DHECsensorcase (Autodesk Fusion 360 design; units mm, degrees)
Autodesk Fusion 360 part; units mm, degrees
sketch "Sketch1" plane through (0, 0, 0) normal (0, 0, 1) x (1, 0, 0)
  line L0 (0, 0) -> (50, 0)
  line L1 (50, 0) -> (50, 39)
  line L2 (50, 39) -> (0, 39)
  line L3 (0, 39) -> (0, 0)
  line L4 (2, 2) -> (48, 2)
  line L5 (48, 2) -> (48, 37)
  line L6 (48, 37) -> (2, 37)
  line L7 (2, 37) -> (2, 2)
  dimension "d1" = 46
  dimension "d2" = 2
  dimension "d3" = 2
  dimension "d4" = 2
  dimension "d5" = 2
  dimension "d6" = 35
  constraint horizontal L0
  constraint vertical L1
  constraint horizontal L2
  constraint vertical L3
  constraint coincident L0.start L3.end
  constraint horizontal L4
  constraint vertical L5
  constraint horizontal L6
  constraint vertical L7
  measures "d1" distance of L5 L7
  measures "d2" distance of L3 L7
  measures "d3" distance of L2 L6
  measures "d4" distance of L0 L4
  measures "d5" distance of L1 L5
  measures "d6" distance of L4 L6
extrude "Extrude1" add sketch "Sketch1" along normal blind 2 contours L4 L5 L6 L7
extrude "Extrude2" add sketch "Sketch1" along normal blind 25
sketch "Sketch2" plane through (50, 0, 0) normal (1, 0, 0) x (0, 1, 0)
  line L0 (0, 0) -> (39, 0)
  line L1 (39, 0) -> (39, 25)
  line L2 (39, 25) -> (0, 25)
  line L3 (0, 25) -> (0, 0)
  line L4 (2, 25) -> (2, 24)
  line L5 (2, 24) -> (1, 24)
  line L6 (1, 24) -> (1, 23)
  line L7 (1, 23) -> (38, 23)
  line L8 (38, 23) -> (38, 24)
  line L9 (38, 24) -> (37, 24)
  line L10 (37, 24) -> (37, 25)
  line L11 (2, 23) -> (37, 23)
  line L12 (37, 23) -> (37, 4)
  line L13 (37, 4) -> (2, 4)
  line L14 (2, 4) -> (2, 23)
  dimension "d11" = 1
  dimension "d12" = 1
  dimension "d13" = 1
  dimension "d14" = 1
  dimension "d15" = 1
  dimension "d16" = 1
  dimension "d17" = 1
  dimension "d18" = 19
  constraint coincident L2 L4.start
  constraint perpendicular L2 L4
  constraint perpendicular L4 L5
  constraint perpendicular L2 L6
  constraint perpendicular L6 L7
  constraint perpendicular L7 L8
  constraint perpendicular L6 L9
  constraint coincident L2 L10.end
  constraint perpendicular L2 L10
  constraint horizontal L11
  constraint vertical L12
  constraint horizontal L13
  constraint vertical L14
  constraint coincident L7 L11.start
  constraint coincident L4.end L14
  constraint coincident L9.end L12
  measures "d11" distance of L2 L5
  measures "d12" distance of L5 L7
  measures "d13" distance of L4 L6
  measures "d14" distance of L3 L6
  measures "d15" distance of L1 L8
  measures "d16" distance of L8 L10
  measures "d17" distance of L7 L9
  measures "d18" distance of L11 L13
extrude "Extrude3" cut sketch "Sketch2" against normal up to surface (48 mm away) contours L2 L4 L5 L6 L7 L8 L9 L10 L11 | L7 L11 L12 L13 L14
sketch "Sketch3" plane through (0, 0, 0) normal (-1, 0, 0) x (0, -1, 0)
  line L0 (-39, 0) -> (0, 0)
  line L1 (0, 0) -> (0, 25)
  line L2 (0, 25) -> (-39, 25)
  line L3 (-39, 25) -> (-39, 0)
  circle A0 centre (-19.5, 12.5) radius 6.75
  circle A1 centre (-19.5, 12.5) radius 4.75
  point P0 (-19.5, 25)
  point P1 (0, 12.5)
  dimension "d21" = 2
  dimension "d22" = 9.5
  constraint concentric A0 A1
  constraint midpoint L2 P0
  constraint midpoint L1 P1
  constraint vertical A0.centre P0
  constraint horizontal A0.centre P1
  measures "d21" distance of A0 A1
  measures "d22" diameter of A1
extrude "Extrude4" add sketch "Sketch3" along normal blind 15 contours A0
